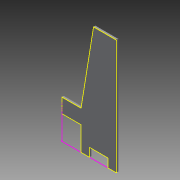
# Autodesk Inventor part: seitenteil
Saved by Autodesk Inventor 2013 (Build 170138000, 138)
## iProperties
Created: 2014-03-27
Part Number: seitenteil
Material: Generic
Document SubType Name: Modeling
Designer: hhanff
Density: 1 g/cm^3
Mass: 8098 g
Surface Area: 8818.1 cm^2
Volume: 8098 cm^3
Author: hhanff
Autodesk Inventor part; units mm, degrees
ref_plane "YZ Plane" through (0, 0, 0) normal (1, 0, 0) x (0, 1, 0)
ref_plane "XZ Plane" through (0, 0, 0) normal (0, 1, 0) x (-1, 0, 0)
ref_plane "XY Plane" through (0, 0, 0) normal (0, 0, 1) x (1, 0, 0)
sketch "Sketch1" plane through (0, 0, 0) normal (0, 1, 0) x (-1, 0, 0)
  line L0 (0, 0) -> (0, 1200)
  line L1 (0, 1200) -> (240, 1200)
  line L2 (370, 400) -> (570, 400)
  line L3 (240, 1200) -> (370, 400)
  line L4 (570, 400) -> (570, 250)
  line L5 (570, 250) -> (370, 250)
  line L6 (370, 0) -> (370, 250)
  line L7 (370, 0) -> (280, 0)
  line L8 (280, 0) -> (280, 90)
  line L9 (280, 90) -> (90, 90)
  line L10 (90, 90) -> (90, 0)
  line L11 (90, 0) -> (0, 0)
  dimension "d2" = 1200
  dimension "d4" = 200
  dimension "d8" = 370
  dimension "d9" = 150
  dimension "d10" = 250
  dimension "d11" = 90
  dimension "d12" = 90
  dimension "d13" = 190
  dimension "d14" = 240
  constraints: 24 end point, 5 perpendicular, 3 parallel, 1 vertical
  measures "d2" distance of L0.start L0.end
  measures "d4" distance of L2.start L2.end
  measures "d8" distance of L0.start L6.start
  measures "d9" distance of L2.end L4.end
  measures "d10" distance of L6.start L5.end
  measures "d11" distance of L6.start L7.end
  measures "d12" distance of L7.end L8.end
  measures "d13" distance of L8.end L9.end
  measures "d14" distance of L0.end L1.end
extrude "Extrusion1" add sketch "Sketch1" along normal blind 20
sketch "Sketch2" plane through (0, 0, 0) normal (0, -1, 0) x (1, 0, 0)
  line L0 (0, 0) -> (0, 1200) projected
  line L1 (0, 1200) -> (-240, 1200) projected
  line L2 (-240, 1200) -> (-240, 400) projected
  line L3 (-370, 400) -> (-570, 400) projected
  line L4 (-570, 400) -> (-570, 0) projected
  line L5 (-570, 0) -> (0, 0) projected
sketch "Sketch3" plane through (0, 0, 0) normal (0, -1, 0) x (1, 0, 0)
  line L0 (0, 0) -> (0, 1200) projected
  line L1 (0, 1200) -> (-240, 1200) projected
  line L2 (-240, 1200) -> (-370, 400) projected
  line L3 (-370, 400) -> (-570, 400) projected
  line L4 (-570, 400) -> (-570, 250) projected
  line L5 (-570, 250) -> (-370, 250) projected
  line L6 (-370, 250) -> (-370, 0) projected
  line L7 (-370, 0) -> (-280, 0) projected
  line L8 (-280, 0) -> (-280, 90) projected
  line L9 (-280, 90) -> (-90, 90) projected
  line L10 (-90, 90) -> (-90, 0) projected
  line L11 (-90, 0) -> (0, 0) projected
sketch "Sketch4" plane through (0, 0, 0) normal (0, -1, 0) x (1, 0, 0)
  line L0 (0, 0) -> (0, 1200) projected
  line L1 (0, 1200) -> (-240, 1200) projected
  line L2 (0, 0) -> (-8, 0)
  line L3 (-8, 0) -> (-8, 1200)
  line L4 (-8, 1200) -> (0, 1200)
  line L5 (0, 1200) -> (0, 0)
  dimension "d15" = 8
  constraints: 8 end point, 2 parallel, 1 horizontal, 1 perpendicular, 1 point on line
  measures "d15" distance of L3.end L4.end
extrude "Extrusion2" cut sketch "Sketch4" against normal blind 10
body "Solid1"
